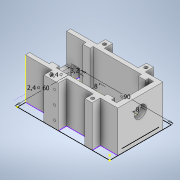
# Autodesk Inventor part: CabezalV1
Saved by Autodesk Inventor 2020.3 (Build 243373000, 373)
## iProperties
Created: 2020-08-25
Part Number: CabezalV1
Material: Generic
Document SubType Name: Modeling
Designer: mifer
Density: 1 g/cm^3
Appearance: Default
Author: mifer
## iProperties of the stored document _3DPrint.ipt
Created: 2020-08-26
Part Number: _3DPrint
Material: Generic
Document SubType Name: Modeling
Designer: mifer
Density: 1 g/cm^3
Appearance: Default
Author: mifer
Autodesk Inventor part; units mm, degrees
ref_plane "YZ Plane" through (0, 0, 0) normal (1, 0, 0) x (0, 1, 0)
ref_plane "XZ Plane" through (0, 0, 0) normal (0, 1, 0) x (-1, 0, 0)
ref_plane "XY Plane" through (0, 0, 0) normal (0, 0, 1) x (1, 0, 0)
sketch "Sketch1" plane through (0, 0, 0) normal (0, 1, 0) x (-1, 0, 0)
  line L0 (0, 0) -> (90, 0)
  line L1 (90, 0) -> (90, -52)
  line L2 (90, -60) -> (0, -60)
  line L3 (0, -60) -> (0, 0)
  line L4 (0, 0) -> (90, 0)
  line L5 (90, 0) -> (90, -8)
  line L6 (90, -8) -> (0, -8)
  line L7 (0, -8) -> (0, 0)
  line L8 (90, -60) -> (0, -60)
  line L9 (0, -60) -> (0, -52)
  line L10 (0, -52) -> (90, -52)
  line L11 (90, -52) -> (90, -60)
  line L12 (0, -8) -> (90, -8)
  line L13 (90, -8) -> (90, -12)
  line L14 (90, -12) -> (0, -12)
  line L15 (0, -12) -> (0, -8)
  line L16 (90, -52) -> (0, -52)
  line L17 (0, -52) -> (0, -48)
  line L18 (0, -48) -> (90, -48)
  line L19 (90, -48) -> (90, -52)
  line L20 (90, 0) -> (64, 0)
  line L21 (64, 0) -> (64, -8)
  line L22 (64, -8) -> (90, -8)
  line L23 (90, -8) -> (90, 0)
  line L24 (64, -8) -> (57, -8)
  line L25 (57, -8) -> (57, 0)
  line L26 (57, 0) -> (64, 0)
  line L27 (64, 0) -> (64, -8)
  line L28 (57, 0) -> (24, 0)
  line L29 (24, 0) -> (24, -8)
  line L30 (24, -8) -> (57, -8)
  line L31 (57, -8) -> (57, 0)
  line L32 (24, -8) -> (17, -8)
  line L33 (17, -8) -> (17, 0)
  line L34 (17, 0) -> (24, 0)
  line L35 (24, 0) -> (24, -8)
  line L36 (57, 0) -> (50, 0)
  line L37 (50, 0) -> (50, -8)
  line L38 (50, -8) -> (57, -8)
  line L39 (57, -8) -> (57, 0)
  line L40 (64, -52) -> (57, -52)
  line L41 (57, -52) -> (57, -60)
  line L42 (57, -60) -> (64, -60)
  line L43 (64, -60) -> (64, -52)
  line L44 (24, -52) -> (17, -52)
  line L45 (17, -52) -> (17, -60)
  line L46 (17, -60) -> (24, -60)
  line L47 (24, -60) -> (24, -52)
  dimension "d0" = 90
  dimension "d1" = 60
  dimension "d49" = 8
  dimension "d50" = 8
  constraints: 96 end point, 24 parallel, 12 horizontal, 12 perpendicular, 12 point on line
  measures "d0" distance of L2.start L2.end
  measures "d1" distance of L0.end L2.start
  measures "d49" distance of L42.end L40.start
  measures "d50" distance of L46.end L44.start
extrude "Extrusion1" add sketch "Sketch1" along normal blind 4 contours L14 L1 L18 L3
extrude "Extrusion2" add sketch "Sketch1" along normal blind 40 contours L0 L29 L6 L33 | L6 L1 L14 L3 | L0 L25 L6 L37 | L18 L1 L10 L3 | L0 L21 L6 L25 | L10 L47 L2 L45 | L43 L2 L41 L10
sketch "Sketch2" plane through (0, 40, 0) normal (0, 1, 0) x (1, 0, 0)
  line L0 (-64, 60) -> (-64, 52) projected
  line L1 (-57, 52) -> (-57, 60) projected
  circle A0 centre (-60.5, 55.5) radius 1.6
  line L2 (-24, 60) -> (-24, 52) projected
  circle A1 centre (-20.5, 56) radius 1.6
  line L3 (-90, 8) -> (-64, 8) projected
  circle A2 centre (-60.5, 4) radius 1.6
  line L4 (-17, 0) -> (-17, 8) projected
  line L5 (-24, 0) -> (-17, 0) projected
  circle A3 centre (-20.5, 4) radius 1.6
  point P0 (0, 0)
  point P1 (-17, 52)
  dimension "d6" = 3.2
  dimension "d7" = 3.2
  dimension "d9" = 3.2
  dimension "d10" = 3.2
  constraints: 4 centre point
  measures "d6" diameter of A0
  measures "d7" diameter of A1
  measures "d9" diameter of A2
  measures "d10" diameter of A3
extrude "Extrusion3" cut sketch "Sketch2" against normal blind 100
sketch "Sketch3" plane through (-64, 0, 0) normal (0, 0, 1) x (1, 0, 0)
  line L0 (0, 0) -> (14, 0) projected
  line L1 (7, 0) -> (7, 40) projected
  line L2 (7, 0) -> (7, 40)
  line L3 (0, 40) -> (14, 40) projected
  circle A0 centre (10.5, 20) radius 1
  circle A1 centre (10.5, 33) radius 1
  circle A2 centre (10.5, 7) radius 1
  point P0 (64, 0)
  dimension "d13" = 2
  constraints: 3 centre point, 2 end point, 1 midpoint, 1 vertical
  measures "d13" diameter of A0
extrude "Extrusion4" cut sketch "Sketch3" against normal blind 30
sketch "Sketch4" plane through (0, 4, 0) normal (0, 1, 0) x (1, 0, 0)
  line L0 (0, 12) -> (-90, 12) projected
  line L1 (0, 48) -> (-90, 48) projected
  line L2 (-90, 12) -> (-86.8, 12)
  line L3 (-86.8, 12) -> (-86.8, 48)
  line L4 (-86.8, 48) -> (-90, 48)
  line L5 (-90, 48) -> (-90, 12)
  line L6 (0, 12) -> (-5, 12)
  line L7 (-5, 12) -> (-5, 48)
  line L8 (-5, 48) -> (0, 48)
  line L9 (0, 48) -> (0, 12)
  line L10 (-17, 12) -> (-10, 12)
  line L11 (-10, 12) -> (-10, 15)
  line L12 (-10, 15) -> (-17, 15)
  line L13 (-17, 15) -> (-17, 12)
  line L14 (-17, 48) -> (-10, 48)
  line L15 (-10, 48) -> (-10, 45)
  line L16 (-10, 45) -> (-17, 45)
  line L17 (-17, 45) -> (-17, 48)
  line L18 (-17, 15) -> (-10, 15)
  line L19 (-10, 21) -> (-17, 21)
  line L20 (-17, 21) -> (-10, 21)
  line L21 (-10, 21) -> (-10, 24)
  line L22 (-10, 24) -> (-17, 24)
  line L23 (-17, 24) -> (-17, 21)
  line L24 (-17, 45) -> (-10, 45)
  line L25 (-10, 39) -> (-17, 39)
  line L26 (-17, 39) -> (-10, 39)
  line L27 (-10, 39) -> (-10, 36)
  line L28 (-10, 36) -> (-17, 36)
  line L29 (-17, 36) -> (-17, 39)
  line L30 (-64, 12) -> (-71, 12)
  line L31 (-71, 12) -> (-71, 15)
  line L32 (-71, 15) -> (-64, 15)
  line L33 (-64, 15) -> (-64, 12)
  line L34 (-64, 21) -> (-71, 21)
  line L35 (-71, 21) -> (-71, 24)
  line L36 (-71, 24) -> (-64, 24)
  line L37 (-64, 24) -> (-64, 21)
  line L38 (-64, 36) -> (-71, 36)
  line L39 (-71, 36) -> (-71, 39)
  line L40 (-71, 39) -> (-64, 39)
  line L41 (-64, 39) -> (-64, 36)
  line L42 (-64, 48) -> (-71, 48)
  line L43 (-71, 48) -> (-71, 45)
  line L44 (-71, 45) -> (-64, 45)
  line L45 (-64, 45) -> (-64, 48)
  line L46 (-10, 48) -> (-17, 48)
  line L47 (-10, 12) -> (-17, 12)
  point P0 (0, 0)
  dimension "d16" = 3.2
  constraints: 92 end point, 22 parallel, 12 horizontal, 10 perpendicular, 7 point on line, 2 collinear
  measures "d16" distance of L4.end L3.end
extrude "Extrusion5" add sketch "Sketch4" along normal blind 36 contours L0 L7 L1 L9
extrude "Extrusion6" add sketch "Sketch4" along normal blind 36 contours L0 L13 L12 L11 | L15 L16 L17 L1 | L0 L31 L32 L33 | L45 L44 L43 L1
extrude "Extrusion7" add sketch "Sketch4" along normal blind 1 contours L19 L23 L22 L21 | L27 L28 L29 L25 | L34 L35 L36 L37 | L38 L39 L40 L41
sketch "Sketch5" plane through (-5, 4, -48) normal (-1, 0, 0) x (0, 0, 1)
  line L0 (0, 36) -> (36, 36) projected
  circle A0 centre (18, 22) radius 6
  point P0 (48, -4)
  constraints: 1 centre point
extrude "Extrusion8" cut sketch "Sketch5" against normal blind 20
sketch "Sketch6" plane through (-90, 0, -8) normal (-1, 0, 0) x (0, 0, 1)
  line L0 (0, 0) -> (-44, 0) projected
  line L1 (-40, 4) -> (-40, 40) projected
  arc A0 (-28, 12) -> (-16, 12) centre (-22, 20) ccw
  line L2 (-37, 4) -> (-37, 40) projected
  line L3 (-4, 12) -> (-16, 12)
  line L4 (-28, 12) -> (-37, 12)
  line L5 (-7, 4) -> (-4, 4) projected
  line L6 (-4, 4) -> (-4, 12)
  line L7 (-4, 40) -> (-4, 4) projected
  line L8 (-40, 4) -> (-4, 4)
  line L9 (-37, 12) -> (-40, 12)
  line L10 (-40, 12) -> (-40, 4)
  point P0 (8, 0)
  dimension "d30" = 20
  constraints: 12 end point, 2 point on circle, 2 point on line, 1 centre point, 1 collinear, 1 perpendicular, 1 vertical
  measures "d30" diameter of A0
extrude "Extrusion9" add sketch "Sketch6" against normal blind 4
sketch "Sketch8" plane through (0, 0, 0) normal (0, -1, 0) x (1, 0, 0)
  line L0 (-64, -52) -> (-90, -52) projected
  line L1 (-86, -52) -> (-76, -52)
  line L2 (-76, -52) -> (-76, -56)
  line L3 (-76, -56) -> (-86, -56)
  line L4 (-86, -56) -> (-86, -52)
  line L5 (-85, -52) -> (-77, -52)
  line L6 (-77, -52) -> (-77, -55)
  line L7 (-77, -55) -> (-85, -55)
  line L8 (-85, -55) -> (-85, -52)
  line L9 (-85, -55) -> (-77, -55)
  line L10 (-77, -55) -> (-77, -46.5727)
  line L11 (-77, -46.5727) -> (-85, -46.5727)
  line L12 (-85, -46.5727) -> (-85, -55)
  point P0 (0, 0)
  constraints: 24 end point, 6 parallel, 3 horizontal, 3 perpendicular, 2 point on line
extrude "Extrusion14" add sketch "Sketch8" against normal blind 15 contours L2 L3 L4 L0 L8 L7 L6 | L6 L7 L8 L0
extrude "Extrusion15" cut sketch "Sketch8" against normal blind 15 contours L6 L7 L8 L0 | L0 L12 L11 L10
sketch "Sketch9" plane through (0, 0, -52) normal (0, 0, -1) x (-1, 0, 0)
  line L0 (0, 0) -> (0, 40) projected
  line L1 (0, 0) -> (36, 0)
  line L2 (36, 0) -> (36, 11.5)
  line L3 (36, 11.5) -> (0, 11.5)
  line L4 (0, 11.5) -> (0, 0)
  circle A0 centre (36, 11.5) radius 1
  dimension "d45" = 11.5
  dimension "d46" = 2
  constraints: 8 end point, 2 parallel, 1 centre point, 1 coincident, 1 horizontal, 1 perpendicular
  measures "d45" distance of L2.end L1.end
  measures "d46" diameter of A0
extrude "Extrusion16" cut sketch "Sketch9" against normal blind 10 contours A0 L2 L3 | L3 L2 A0
sketch "Sketch10" plane through (-90, 0, -8) normal (-1, 0, 0) x (0, 0, 1)
  line L0 (-44, 0) -> (-52, 0) projected
  line L1 (-44, 0) -> (-44, 7)
  line L2 (-44, 0) -> (-44, 40) projected
  circle A0 centre (-33, 7) radius 1.2
  line L3 (0, 0) -> (0, 40) projected
  line L4 (0, 7) -> (11, 7) construction
  circle A1 centre (-11, 7) radius 1.2
  point P0 (8, 0)
  dimension "d51" = 2.4
  dimension "d54" = 2.4
  constraints: 4 end point, 2 centre point, 2 point on line, 1 horizontal
  measures "d51" diameter of A0
  measures "d54" diameter of A1
body "Solid1"
